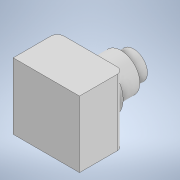
# Autodesk Inventor part: Practica 12 nt
Saved by Autodesk Inventor 2020.2 (Build 242310000, 310)
## iProperties
Created: 2020-02-28
Part Number: Practica 12 nt
Material: Genérico
Document SubType Name: Chapa
Designer: Luis Gallardo
Density: 1 g/cm^3
Sheet Metal Rule: Por defecto_mm
Appearance: Valor por defecto
Author: Luis Gallardo
Autodesk Inventor part; units mm, degrees
ref_plane "YZ Plane" through (0, 0, 0) normal (1, 0, 0) x (0, 1, 0)
ref_plane "XZ Plane" through (0, 0, 0) normal (0, 1, 0) x (-1, 0, 0)
ref_plane "XY Plane" through (0, 0, 0) normal (0, 0, 1) x (1, 0, 0)
sketch "Boceto1" plane through (0, 0, 0) normal (0, 1, 0) x (-1, 0, 0)
  line L0 (0, 0) -> (-60, 0)
  line L1 (-60, 0) -> (-60, -34)
  line L2 (-54, -40) -> (-6, -40)
  line L3 (0, -34) -> (0, 0)
  arc A0 (-6, -40) -> (0, -34) centre (-6, -34) ccw
  arc A1 (-60, -34) -> (-54, -40) centre (-54, -34) ccw
  point P0 (-60, -40)
  dimension "d0" = 60
  dimension "d1" = 40
  dimension "d2" = 6
  dimension "d3" = 6
  constraints: 8 end point, 4 point on circle, 4 tangent, 3 perpendicular, 2 centre point, 2 point on line, 1 horizontal
  measures "d0" distance of L0.start L0.end
  measures "d1" distance of L0.end point (-60, -40)
  measures "d2" radius of A0
  measures "d3" radius of A1
extrude "Extrusión1" add sketch "Boceto1" along normal blind 60
sketch "Boceto2" plane through (54, 0, -40) normal (0, 0, -1) x (-1, 0, 0)
  line L0 (0, 0) -> (48, 0) projected
  line L1 (48, 0) -> (48, 60) projected
  line L2 (0, 60) -> (48, 60) projected
  line L3 (0, 0) -> (0, 60) projected
  circle A0 centre (24, 30) radius 22.5
  circle A1 centre (24, 30) radius 17
  circle A2 centre (24, 30) radius 15
  circle A3 centre (24, 30) radius 12.5
  point P0 (54, 0)
  dimension "d6" = 45
  dimension "d7" = 34
  dimension "d8" = 30
  dimension "d9" = 25
  constraints: 4 centre point, 3 coincident
  measures "d6" diameter of A0
  measures "d7" diameter of A1
  measures "d8" diameter of A2
  measures "d9" diameter of A3
extrude "Extrusión3" add sketch "Boceto2" along normal blind 7 contours A0
sketch "Boceto5" plane through (30, 30, -40) normal (0, 0, -1) x (-1, 0, 0)
  circle A0 centre (0, 0) radius 17
  point P0 (30, -30)
  dimension "d14" = 34
  constraints: 1 centre point
  measures "d14" diameter of A0
extrude "Extrusión4" add sketch "Boceto5" along normal blind 27.59
fillet "Empalme1" radius 2 1 edges at (47, 30, -47)
sketch "Boceto8" plane through (30, 30, -67.59) normal (0, 0, -1) x (-1, 0, 0)
  circle A0 centre (0, 0) radius 12.5
  point P0 (30, -30)
  dimension "d23" = 25
  constraints: 1 centre point
  measures "d23" diameter of A0
extrude "Extrusión6" add sketch "Boceto8" along normal blind 11.41
sketch "Boceto9" plane through (30, 30, -79) normal (0, 0, -1) x (-1, 0, 0)
  point P0 (30, -30)
equation "\"Radio_pliegue\" = Grosor"
equation "\"Anchura_desahogo_plegado\" = Grosor"
equation "\"Profundidad_desahogo_plegado\" = 0.5 * Grosor"
equation "\"Tamaño_destalonado\" = 4 * Grosor"
equation "\"Remanente_mínimo\" = 2 * Grosor"
equation "\"Radiodetransición\" = Radio_pliegue"
equation "\"Tamaño_de_radio_de_Jacobi\" = Radio_pliegue"
equation "\"TamañoSeparación\" = Grosor"
equation "\"Grosor\" = 0.5"
